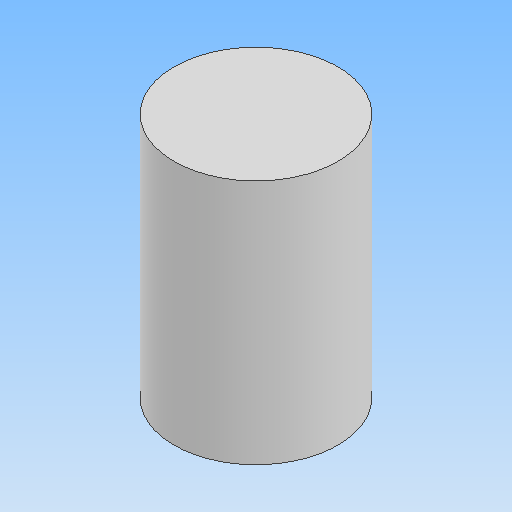
# Autodesk Inventor part: Cylinder-sizing (plug-demo1)
Saved by Autodesk Inventor 2026.1 (Build 301233020, 233B)
## iProperties
Created: 2026-02-13
Part Number: Cylinder-sizing (plug-demo1)
Material: Generic
Document SubType Name: Modeling
Designer: holy
Density: 1 g/cm^3
Appearance: Default
Author: holy
Autodesk Inventor part; units mm, degrees
ref_plane "YZ Plane" through (0, 0, 0) normal (1, 0, 0) x (0, 1, 0)
ref_plane "XZ Plane" through (0, 0, 0) normal (0, 1, 0) x (-1, 0, 0)
ref_plane "XY Plane" through (0, 0, 0) normal (0, 0, 1) x (1, 0, 0)
sketch "Sketch1" plane through (0, 0, 0) normal (0, 1, 0) x (-1, 0, 0)
  line L0 (711.2, 0) -> (-711.2, 0) construction
  line L1 (0, -711.2) -> (0, 711.2) construction
  circle A0 centre (0, 0) radius 200
  dimension "d0" = 400
  constraints: 1 centre point, 1 coincident
  measures "d0" diameter of A0
extrude "Extrusion1" add sketch "Sketch1" along normal blind 600
equation "\"d0\" = Dia"
equation "\"d1\" = Height"
equation "\"Dia\" = 400"
equation "\"Height\" = 600"
body "Solid1"
